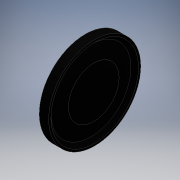
# Autodesk Inventor part: ET20
Saved by Autodesk Inventor 2016 (Build 200138000, 138)
## iProperties
Created: 2016-03-28
Part Number: ET20
Material: Genérico
Document SubType Name: Modeling
Designer: Usuario1
Density: 1 g/cm^3
Appearance: Valor por defecto
Author: Usuario1
Autodesk Inventor part; units mm, degrees
ref_plane "YZ Plane" through (0, 0, 0) normal (1, 0, 0) x (0, 1, 0)
ref_plane "XZ Plane" through (0, 0, 0) normal (0, 1, 0) x (-1, 0, 0)
ref_plane "XY Plane" through (0, 0, 0) normal (0, 0, 1) x (1, 0, 0)
sketch "Boceto1" plane through (0, 0, 0) normal (1, 0, 0) x (0, 1, 0)
  circle A0 centre (0, -0.0022) radius 0.8492
  circle A1 centre (0, 0) radius 0.9775
  circle A2 centre (0, 0) radius 0.925
  dimension "d1" = 1.85
  constraints: 3 centre point
  measures "d1" diameter of A2
extrude "Extrusión1" add sketch "Boceto1" along normal blind 0.1 contours A1
sketch "Boceto2" plane through (0, 0, 0) normal (1, 0, 0) x (0, 1, 0)
  circle A0 centre (0, -0.0022) radius 0.8492
  circle A1 centre (0, 0) radius 0.9775
  circle A2 centre (0, 0) radius 0.925 projected
  constraints: 2 centre point
extrude "Extrusión2" add sketch "Boceto2" along normal blind 0.1 contours A2
chamfer "Chaflán1" distance 0.08 angle 45 1 edges at (0.1, -0.8492, -0.0022)
sketch "Boceto3" plane through (0, 0, 0) normal (1, 0, 0) x (0, 1, 0)
  circle A0 centre (0, -0.0022) radius 0.8492 projected
  point P0 (0, 0)
extrude "Extrusión3" add sketch "Boceto3" along normal blind 0.08
fillet "Empalme1" radius 0.84 1 edges at (0.08, -0.8492, -0.0022)
sketch "Boceto4" plane through (0, 0, 0) normal (-1, 0, 0) x (0, 0, 1)
  line L0 (-0.8864, -0.025) -> (-0.9364, -0.025)
  line L1 (-0.9364, -0.025) -> (-0.9364, 0.025)
  line L2 (-0.9364, 0.025) -> (-0.8864, 0.025)
  line L3 (-0.8864, 0.025) -> (-0.8864, -0.025)
  line L4 (0.8864, 0.025) -> (0.9364, 0.025)
  line L5 (0.9364, 0.025) -> (0.9364, -0.025)
  line L6 (0.9364, -0.025) -> (0.8864, -0.025)
  line L7 (0.8864, -0.025) -> (0.8864, 0.025)
  circle A0 centre (0, 0) radius 0.9775
  constraints: 16 end point, 1 centre point
extrude "Extrusión4" add sketch "Boceto4" along normal blind 0.1 contours L0 L1 L2 L3 | L4 L5 L6 L7
sketch "Boceto5" plane through (0, 0, 0) normal (-1, 0, 0) x (0, 0, 1)
  line L0 (-0.9364, -0.025) -> (-0.9364, 0.025) projected
  line L1 (-0.9364, 0.025) -> (-0.8864, 0.025) projected
  line L2 (-0.8864, 0.025) -> (-0.8864, -0.025) projected
  line L3 (-0.8864, -0.025) -> (-0.9364, -0.025) projected
  line L4 (0.9364, 0.025) -> (0.9364, -0.025) projected
  line L5 (0.9364, -0.025) -> (0.8864, -0.025) projected
  line L6 (0.8864, -0.025) -> (0.8864, 0.025) projected
  line L7 (0.8864, 0.025) -> (0.9364, 0.025) projected
  circle A0 centre (0, 0) radius 0.9775 projected
extrude "Extrusión5" add sketch "Boceto5" along normal blind 0.1
